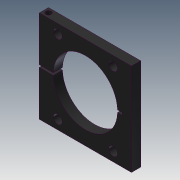
# Autodesk Inventor part: JF-AT-JC0015
Saved by Autodesk Inventor 2015 SP1 (Build 190203100, 203)
## iProperties
Created: 2010-04-29
Part Number: JF-AT-JC0015
Document SubType Name: Modeling
Designer: InventorUser
Density: 2.71 g/cm^3
Material: Aluminum-6061 (Anodized Black)
Description: Can Clamp
Mass: 39.0618 g
Surface Area: 84.2467 cm^2
Volume: 14.4139 cm^3
Vendor: HHMI: JRC -ID&F
Appearance: Metal-AL-6061 (anodized black)
Revision Number: 0
Autodesk Inventor part; units mm, degrees
ref_plane "YZ Plane" through (0, 0, 0) normal (1, 0, 0) x (0, 1, 0)
ref_plane "XZ Plane" through (0, 0, 0) normal (0, 1, 0) x (-1, 0, 0)
ref_plane "XY Plane" through (0, 0, 0) normal (0, 0, 1) x (1, 0, 0)
sketch "Sketch1" plane through (0, 0, 0) normal (0, 0, 1) x (1, 0, 0)
  line L0 (-16.2013, 52.9706) -> (47.2987, 52.9706)
  line L1 (47.2987, 52.9706) -> (47.2987, -10.5294)
  line L2 (47.2987, -10.5294) -> (-16.2013, -10.5294)
  line L3 (-16.2013, -10.5294) -> (-16.2013, 52.9706)
  point P0 (0, 0)
  dimension "d0" = 63.5
  dimension "d1" = 63.5
  constraints: 8 end point
  measures "d0" distance between parallel lines of L2 L0
  measures "d1" distance between parallel lines of L1 L3
extrude "Extrusion1" add sketch "Sketch1" along normal blind 6.35
sketch "Sketch2" plane through (0, 0, 6.35) normal (0, 0, 1) x (1, 0, 0)
  line L0 (-16.2013, -10.5294) -> (-16.2013, 52.9706) projected
  line L1 (47.2987, -10.5294) -> (-16.2013, -10.5294) projected
  point P0 (0, 0)
  point P1 (15.5487, 21.2206)
  dimension "d4" = 31.75
  dimension "d5" = 31.75
  measures "d4" distance from line of L0 point (15.549, 21.221)
  measures "d5" distance from line of L1 point (15.549, 21.221)
hole "Hole1" at (15.5487, 21.2206, 6.35) direction (0, 0, -1) diameter 44.323 end through all
sketch "Sketch3" plane through (0, 0, 6.35) normal (0, 0, 1) x (1, 0, 0)
  line L0 (47.2987, 52.9706) -> (47.2987, -10.5294) projected
  line L1 (-16.2013, 52.9706) -> (47.2987, 52.9706) projected
  line L2 (-16.2013, -10.5294) -> (-16.2013, 52.9706) projected
  line L3 (47.2987, -10.5294) -> (-16.2013, -10.5294) projected
  point P0 (0, 0)
  point P1 (-3.5013, 46.6206)
  point P2 (34.5987, 46.6206)
  point P3 (-3.5013, -4.1794)
  point P4 (34.5987, -4.1794)
  dimension "d13" = 6.35
  dimension "d14" = 12.7
  dimension "d15" = 12.7
  dimension "d16" = 6.35
  dimension "d24" = 12.7
  dimension "d25" = 12.7
  measures "d13" distance from line of L1 point (-3.501, 46.621)
  measures "d14" distance from line of L2 point (-3.501, 46.621)
  measures "d15" distance from line of L0 point (34.599, 46.621)
  measures "d16" distance from line of L3 point (-3.501, -4.179)
  measures "d24" distance from line of L2 point (-3.501, -4.179)
  measures "d25" distance from line of L0 point (34.599, -4.179)
hole "Hole2" at (-3.5013, 46.6206, 6.35) at (34.5987, 46.6206, 6.35) at (-3.5013, -4.1794, 6.35) at (34.5987, -4.1794, 6.35) direction (0, 0, -1) diameter 6.096 end through all
sketch "Sketch4" plane through (0, 0, 6.35) normal (0, 0, 1) x (1, 0, 0)
  line L0 (-16.2013, 52.9706) -> (47.2987, 52.9706) projected
  line L1 (-4.7209, 20.4332) -> (-21.033, 20.4332)
  line L2 (-21.033, 20.4332) -> (-21.033, 22.0207)
  line L3 (-21.033, 22.0207) -> (-4.7209, 22.0207)
  line L4 (-4.7209, 22.0207) -> (-4.7209, 20.4332)
  point P0 (0, 0)
  dimension "d26" = 1.5875
  dimension "d27" = 30.9499
  constraints: 8 end point
  measures "d26" distance between parallel lines of L1 L3
  measures "d27" distance between parallel lines of L3 L0
extrude "Extrusion2" cut sketch "Sketch4" against normal blind 6.35
sketch "Sketch5" plane through (-16.2013, 52.9706, 0) normal (0, 1, 0) x (1, 0, 0)
  line L0 (0, 0) -> (63.5, 0) projected
  line L1 (0, 0) -> (0, -6.35) projected
  point P0 (16.2013, 0)
  point P1 (3.175, -3.175)
  dimension "d30" = 3.175
  dimension "d31" = 3.175
  measures "d30" distance from line of L0 point (3.175, -3.175)
  measures "d31" distance from line of point (3.175, -3.175) L1
hole "Hole3" at (-13.0263, 52.9706, 3.175) direction (0, -1, 0) diameter 2.6416 depth 50.8 tip angle 118 thread size "6-32 UNC" class "2B" standard "ANSI Unified Screw Threads"
sketch "Sketch6" plane through (-16.2013, 52.9706, 0) normal (0, 1, 0) x (1, 0, 0)
  circle A0 centre (3.175, -3.175) radius 1.3208 projected
  point P0 (16.2013, 0)
  constraints: 1 coincident
hole "Hole4" at (-13.0263, 52.9706, 3.175) direction (0, -1, 0) diameter 3.81 depth 31.75 tip angle 118
sketch "Sketch7" plane through (0, 0, 0) normal (0, 0, -1) x (-1, 0, 0)
  line L0 (-47.2987, 52.9706) -> (-47.2987, -10.5294) projected
  line L1 (-40.9487, 22.0207) -> (-35.1672, 22.0207)
  line L2 (-35.1672, 22.0207) -> (-35.1672, 20.4332)
  line L3 (-35.1672, 20.4332) -> (-40.9487, 20.4332)
  line L4 (-40.9487, 20.4332) -> (-40.9487, 22.0207)
  point P0 (0, 0)
  dimension "d46" = 6.35
  constraints: 8 end point
  measures "d46" distance from line of L0 L1.start
extrude "Extrusion3" cut sketch "Sketch7" against normal blind 6.35
body "Solid1"
